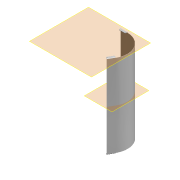
# Autodesk Inventor part: Part26
Saved by Autodesk Inventor 2014 (Build 180170000, 170)
## iProperties
Created: 2016-03-29
Part Number: Part26
Material: Aluminum 6061
Document SubType Name: Modeling
Designer: admin
Density: 1 g/cm^3
Appearance: Smooth - White
Author: admin
Autodesk Inventor part; units mm, degrees
ref_plane "YZ Plane" through (0, 0, 0) normal (1, 0, 0) x (0, 1, 0)
ref_plane "XZ Plane" through (0, 0, 0) normal (0, 1, 0) x (-1, 0, 0)
ref_plane "Work Plane1" through (0, 0, 0) normal (0, 0, 1) x (1, 0, 0)
sketch "Sketch1" plane through (0, 0, 0) normal (0, 0, 1) x (1, 0, 0)
  arc A0 (173.074137, -21.982113) -> (67.5, 160.877656) centre (67.5, 38.971143) ccw
  line L0 (67.5, 160.877656) -> (23, 160.877656)
  line L1 (150.824137, -60.520244) -> (173.074137, -21.982113)
  line L2 (23, 162.377656) -> (67.5, 162.377656)
  arc A1 (174.373175, -22.732113) -> (67.5, 162.377656) centre (67.5, 38.971143) ccw
  line L3 (174.373175, -22.732113) -> (152.123175, -61.270244)
  line L4 (150.824137, -60.520244) -> (152.123175, -61.270244)
  line L5 (23, 160.877656) -> (23, 162.377656)
  point P0 (0, 0)
  dimension "d0" = 1.5
  constraints: 8 end point, 2 perpendicular, 2 point on circle, 1 centre point, 2 other
  measures "d0" radial gap between concentric circles of A1 A0
ref_plane "Work Plane2" through (-342.433406, -360.707407, -533) normal (0, 0, -1) x (0, 1, 0)
extrude "Extrusion1" add sketch "Sketch1" against normal blind 551
sketch "Sketch2" plane through (0, 0, 0) normal (0, 0, 1) x (1, 0, 0)
  line L0 (174.373175, -22.732113) -> (152.123175, -61.270244)
  arc A0 (174.373175, -22.732113) -> (67.5, 162.377656) centre (67.5, 38.971143) ccw
  line L1 (23, 162.377656) -> (67.5, 162.377656)
  line L2 (23, 162.377656) -> (67.5, 162.377656)
  line L3 (67.5, 162.377656) -> (67.5, 147.377656)
  line L4 (67.5, 147.377656) -> (23, 147.377656)
  line L5 (23, 147.377656) -> (23, 162.377656)
  line L6 (152.123175, -61.270244) -> (174.373175, -22.732113)
  line L7 (174.373175, -22.732113) -> (161.382794, -15.232113)
  line L8 (161.382794, -15.232113) -> (139.132794, -53.770244)
  line L9 (139.132794, -53.770244) -> (152.123175, -61.270244)
  point P0 (0, 0)
  dimension "d3" = 15
  dimension "d4" = 15
  constraints: 16 end point, 6 equal length, 2 perpendicular, 2 tangent
  measures "d3" distance of L1.end L3.end
  measures "d4" distance of L7.end L0.start
extrude "Extrusion2" add sketch "Sketch2" along normal blind 1.5
fillet "Fillet4" radius 6 4 edges at (161.3828, -15.2321, 0.75) (139.1328, -53.7702, 0.75) (23, 147.3777, 0.75) (67.5, 147.3777, 0.75)
sketch "Sketch5" plane through (0, 0, 1.5) normal (0, 0, 1) x (1, 0, 0)
  arc A0 (61.5, 147.377656) -> (67.5, 153.377656) centre (61.5, 153.377656) ccw
  arc A1 (23, 153.377656) -> (29, 147.377656) centre (29, 153.377656) ccw
  arc A2 (142.132794, -48.574091) -> (144.328946, -56.770244) centre (147.328946, -51.574091) ccw
  line L0 (144.328946, -56.770244) -> (152.123175, -61.270244)
  line L1 (174.373175, -22.732113) -> (166.578946, -18.232113)
  arc A3 (166.578946, -18.232113) -> (158.382794, -20.428266) centre (163.578946, -23.428266) ccw
  line L2 (158.382794, -20.428266) -> (142.132794, -48.574091)
  circle A4 centre (29, 153.377656) radius 2
  circle A5 centre (61.5, 153.377656) radius 2
  circle A6 centre (163.578946, -23.428266) radius 2
  circle A7 centre (147.328946, -51.574091) radius 2
  line L3 (152.123175, -61.270244) -> (174.373175, -22.732113)
  point P0 (0, 0)
  dimension "d17" = 4
  dimension "d18" = 4
  dimension "d19" = 4
  dimension "d20" = 4
  constraints: 4 centre point, 4 coincident
  measures "d17" diameter of A4
  measures "d18" diameter of A5
  measures "d19" diameter of A6
  measures "d20" diameter of A7
extrude "Extrusion5" cut sketch "Sketch5" against normal blind 2 contours A4 | A5 | A6 | A7
fillet "Fillet5" radius 1.5 2 edges at (45.25, 160.8777, 0) (161.9491, -41.2512, 0)
ref_plane "Work Plane5" through (0, 0, -275.5) normal (0, 0, 1) x (1, 0, 0)
mirror "Mirror3" about plane through (0, 0, -275.5) normal (0, 0, 1) of "Extrusion2", "Extrusion5", "Fillet4", "Fillet5"
sketch "Sketch7" plane through (0, 0, -551) normal (0, 0, -1) x (-1, 0, 0)
  line L0 (-67.5, 160.877656) -> (-67.5, 162.377656)
  arc A0 (-67.5, 162.377656) -> (-174.373175, -22.732113) centre (-67.5, 38.971143) ccw
  line L1 (-174.373175, -22.732113) -> (-173.074137, -21.982113)
  arc A1 (-67.5, 160.877656) -> (-173.074137, -21.982113) centre (-67.5, 38.971143) ccw
  point P0 (0, 0)
extrude "Extrusion7" cut sketch "Sketch7" against normal blind 2
sketch "Sketch8" plane through (0, 0, 0) normal (0, 0, 1) x (1, 0, 0)
  line L0 (67.5, 162.377656) -> (67.5, 160.877656)
  arc A0 (173.074137, -21.982113) -> (67.5, 160.877656) centre (67.5, 38.971143) ccw
  line L1 (173.074137, -21.982113) -> (174.373175, -22.732113)
  arc A1 (174.373175, -22.732113) -> (67.5, 162.377656) centre (67.5, 38.971143) ccw
  point P0 (0, 0)
extrude "Extrusion8" cut sketch "Sketch8" against normal blind 2
fillet "Fillet7" radius 3 4 edges at (45.25, 162.3777, 1.5) (163.2482, -42.0012, 1.5) (163.2482, -42.0012, -552.5) (45.25, 162.3777, -552.5)
body "Solid1"
